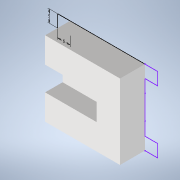
# Autodesk Inventor part: PotiHalterungUnten
Saved by Autodesk Inventor 2020.3 (Build 243373010, 373A)
## iProperties
Created: 2020-11-30
Part Number: PotiHalterungUnten
Material: Generisch
Document SubType Name: Modeling
Designer: Stefan
Density: 1 g/cm^3
Appearance: Vorgabe
Author: Stefan
Autodesk Inventor part; units mm, degrees
ref_plane "YZ Plane" through (0, 0, 0) normal (1, 0, 0) x (0, 1, 0)
ref_plane "XZ Plane" through (0, 0, 0) normal (0, 1, 0) x (-1, 0, 0)
ref_plane "XY Plane" through (0, 0, 0) normal (0, 0, 1) x (1, 0, 0)
sketch "Skizze1" plane through (0, 0, 0) normal (0, 0, 1) x (1, 0, 0)
  line L0 (-15, 15) -> (15, 15)
  line L1 (15, 15) -> (15, -15)
  line L2 (15, -15) -> (-15, -15)
  line L3 (-15, 4.8) -> (5.6, 4.8)
  line L4 (5.6, 4.8) -> (5.6, -4.8)
  line L5 (5.6, -4.8) -> (-15, -4.8)
  line L6 (-15, -15) -> (-15, -4.8)
  line L7 (-15, 4.8) -> (-15, 15)
  point P0 (0, 0)
  dimension "d0" = 30
  dimension "d1" = 30
  dimension "d2" = 15
  dimension "d3" = 15
  dimension "d4" = 9.6
  dimension "d5" = 4.8
  dimension "d6" = 5.6
  constraints: 16 end point, 4 parallel, 2 horizontal, 2 perpendicular
  measures "d0" distance of L1.end L2.end
  measures "d1" distance of L0.end L1.end
  measures "d2" distance from line of point (0, 0) L1
  measures "d3" distance from line of L0 point (0, 0)
  measures "d4" distance of L3.end L4.end
  measures "d5" distance from line of L3 point (0, 0)
  measures "d6" distance from line of point (0, 0) L4
extrude "Extrusion1" add sketch "Skizze1" along normal blind 7
sketch "Skizze2" plane through (0, 0, 0) normal (0, 0, -1) x (-1, 0, 0)
  line L0 (15, -15) -> (-15, -15) projected
  line L1 (15, -15) -> (-15, -15)
  line L2 (-15, -15) -> (-15, 15)
  line L3 (-15, 15) -> (15, 15)
  line L4 (15, 15) -> (15, -15)
  point P0 (0, 0)
  constraints: 8 end point, 2 parallel, 1 horizontal, 1 perpendicular
extrude "Extrusion2" add sketch "Skizze2" along normal blind 3
sketch "Skizze3" plane through (0, 0, -3) normal (0, 0, -1) x (-1, 0, 0)
  line L0 (-15, 15) -> (15, 15) projected
  line L1 (-15, 15) -> (15, 15)
  line L2 (15, 10) -> (15, -10)
  line L3 (15, -15) -> (-15, -15)
  line L4 (15, 15) -> (20, 15)
  line L5 (20, 15) -> (20, 10)
  line L6 (20, 10) -> (15, 10)
  line L7 (-15, 0) -> (15, 0) construction
  line L8 (15, -4.8) -> (15, 4.8) projected
  line L9 (15, -15) -> (-15, -15) projected
  line L10 (0, -15) -> (0, 15) construction
  line L11 (15, -15) -> (20, -15)
  line L12 (20, -15) -> (20, -10)
  line L13 (20, -10) -> (15, -10)
  line L14 (-15, 15) -> (-20, 15)
  line L15 (-20, 15) -> (-20, 10)
  line L16 (-20, 10) -> (-15, 10)
  line L17 (-15, -10) -> (-15, 10)
  line L18 (-15, -15) -> (-20, -15)
  line L19 (-20, -15) -> (-20, -10)
  line L20 (-20, -10) -> (-15, -10)
  point P0 (0, 0)
  point P1 (15, -15)
  point P2 (-15, 15)
  point P3 (-15, -4.8)
  point P4 (-15, 4.8)
  point P5 (-15, -15)
  point P6 (-15, -15)
  dimension "d11" = 5
  dimension "d12" = 5
  constraints: 36 end point, 17 symmetric about line, 3 midpoint, 2 horizontal, 2 parallel, 2 perpendicular, 2 point on line
  measures "d11" distance of L2.start L5.end
  measures "d12" distance of L4.end L5.end
extrude "Extrusion3" add sketch "Skizze3" along normal blind 4
